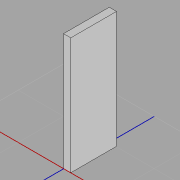
# Autodesk Inventor part: внутр
Saved by Autodesk Inventor 2022 (Build 260153000, 153)
## iProperties
Created: 2022-04-10
Part Number: внутр
Material: Типовые
Document SubType Name: Modeling
Designer: A
Density: 1 g/cm^3
Appearance: По умолчанию
Author: A
Autodesk Inventor part; units mm, degrees
ref_plane "YZ Plane" through (0, 0, 0) normal (1, 0, 0) x (0, 1, 0)
ref_plane "XZ Plane" through (0, 0, 0) normal (0, 1, 0) x (-1, 0, 0)
ref_plane "XY Plane" through (0, 0, 0) normal (0, 0, 1) x (1, 0, 0)
sketch "Эскиз2" plane through (0, 0, 0) normal (1, 0, 0) x (0, 1, 0)
  line L0 (0, 0) -> (258, 0)
  line L1 (258, 0) -> (258, -101)
  line L2 (258, -101) -> (0, -101)
  line L3 (0, -101) -> (0, 0)
  dimension "d4" = 258
  dimension "d5" = 101
  constraints: 8 end point, 2 parallel, 1 horizontal, 1 perpendicular
  measures "d4" distance of L1.end L2.end
  measures "d5" distance of L0.end L1.end
extrude "Выдавливание2" add sketch "Эскиз2" along normal blind 16
